Autodesk Fusion 360 part; units mm, degrees
(part 2 of 3)
sketch "gears_laser_cut" plane through (0, 0, 0) normal (1, 0, 0) x (0, 0, -1)
  arc A0 (348.8153, 272.0785) -> (348.6305, 272.3491) centre (348.5669, 272.1073) ccw
  arc A1 (349.0339, 271.6922) -> (348.78, 271.7745) centre (344.1421, 257.037) ccw
  arc A2 (342.0659, 272.3469) -> (341.8017, 272.3087) centre (344.1421, 257.037) ccw
  arc A3 (345.287, 272.746) -> (345.0457, 272.9677) centre (345.0386, 272.7178) ccw
  arc A4 (347.0702, 272.5131) -> (346.8558, 272.7609) centre (346.8202, 272.5134) ccw
  line L0 (365.4314, 255.9231) -> (365.9486, 256.0584)
  line L1 (387.4886, 271.4519) -> (387.367, 270.9313)
  line L2 (387.305, 271.7538) -> (387.3359, 271.7418)
  line L3 (348.5984, 272.3575) -> (347.7859, 272.5711)
  line L4 (365.2501, 255.6199) -> (365.3445, 254.7966)
  line L5 (365.4024, 256.3282) -> (365.9379, 256.2419)
  line L6 (343.1909, 272.964) -> (343.2239, 272.9669)
  line L7 (369.0501, 267.4461) -> (368.5255, 266.8046)
  line L8 (386.5329, 272.0545) -> (386.4983, 272.0679)
  line L9 (370.3154, 268.7566) -> (370.3392, 268.7797)
  arc A5 (382.3711, 241.8617) -> (382.5542, 241.8777) centre (381.1421, 257.037) ccw
  arc A6 (349.4983, 272.0679) -> (349.1921, 271.9615) centre (349.4076, 271.8349) ccw
  line L10 (365.1921, 257.4407) -> (365.1921, 256.612)
  arc A7 (343.4888, 272.7741) -> (343.2239, 272.9669) centre (343.2452, 272.7178) ccw
  arc A8 (349.2026, 242.1214) -> (349.5112, 242.0112) centre (349.4205, 242.2441) ccw
  arc A9 (345.341, 241.6336) -> (345.6069, 241.6566) centre (344.1421, 257.037) ccw
  line L11 (387.8604, 271.2886) -> (387.5342, 270.8552)
  arc A10 (345.5874, 272.4193) -> (345.3215, 272.4419) centre (344.1421, 257.037) ccw
  arc A11 (382.0595, 241.1067) -> (382.3002, 241.324) centre (382.0523, 241.3566) ccw
  arc A12 (346.8694, 241.3151) -> (347.0838, 241.5584) centre (346.8338, 241.5626) ccw
  arc A13 (340.3342, 272.0104) -> (340.0761, 271.9424) centre (344.1421, 257.037) ccw
  line L12 (369.6642, 267.8305) -> (369.9756, 267.3863)
  arc A14 (342.3169, 272.889) -> (342.0889, 272.6584) centre (342.3382, 272.6399) ccw
  arc A15 (341.6992, 272.5971) -> (341.414, 272.7584) centre (341.4636, 272.5133) ccw
  arc A16 (340.5218, 272.5776) -> (340.3216, 272.3225) centre (340.5714, 272.3326) ccw
  arc A17 (344.1357, 272.9937) -> (343.883, 272.7906) centre (344.1286, 272.7438) ccw
  line L13 (370.3154, 268.7566) -> (369.7212, 268.1791)
  line L14 (388.2096, 271.3421) -> (388.1768, 271.3594)
  arc A18 (348.7987, 242.3055) -> (349.0524, 242.3881) centre (344.1421, 257.037) ccw
  line L15 (348.5984, 272.3575) -> (348.6305, 272.3491)
  arc A19 (380.9075, 241.2886) -> (381.161, 241.0811) centre (381.1539, 241.331) ccw
  line L16 (347.4579, 272.4399) -> (347.3315, 272.1543)
  arc A20 (345.9547, 272.8904) -> (345.6805, 272.7174) centre (345.9191, 272.643) ccw
  arc A21 (347.75, 272.5805) -> (347.4579, 272.4399) centre (347.6865, 272.3387) ccw
  arc A22 (384.0929, 242.1007) -> (384.273, 242.1374) centre (381.1421, 257.037) ccw
  arc A23 (384.4805, 241.6447) -> (384.7745, 241.5) centre (384.7109, 241.7418) ccw
  arc A24 (347.4694, 241.6418) -> (347.7633, 241.4971) centre (347.6998, 241.7389) ccw
  arc A25 (382.7042, 241.3645) -> (382.9797, 241.1872) centre (382.9442, 241.4347) ccw
  line L17 (369.7212, 268.1791) -> (369.6946, 268.1533)
  line L18 (343.883, 272.7906) -> (343.8246, 272.4838)
  line L19 (369.3939, 267.5274) -> (369.8514, 267.2508)
  arc A26 (380.2376, 241.106) -> (380.5015, 241.2944) centre (380.2589, 241.3551) ccw
  line L20 (341.3815, 272.7518) -> (341.414, 272.7584)
  line L21 (369.0501, 267.4461) -> (369.071, 267.4717)
  line L22 (347.0838, 241.5584) -> (347.089, 241.8707)
  line L23 (387.305, 271.7538) -> (386.5329, 272.0545)
  arc A27 (343.8246, 272.4838) -> (343.5578, 272.476) centre (344.1421, 257.037) ccw
  line L24 (345.0126, 272.9687) -> (345.0457, 272.9677)
  arc A28 (347.3315, 272.1543) -> (347.0698, 272.2071) centre (344.1421, 257.037) ccw
  arc A29 (345.0595, 241.1067) -> (345.3002, 241.324) centre (345.0523, 241.3566) ccw
  line L25 (348.608, 241.7191) -> (348.6438, 241.7285)
  line L26 (365.2501, 255.6199) -> (365.2463, 255.6528)
  line L27 (384.8065, 241.5084) -> (384.7745, 241.5)
  arc A30 (347.089, 241.8707) -> (347.3506, 241.9238) centre (344.1421, 257.037) ccw
  arc A31 (339.9414, 272.2172) -> (339.6397, 272.3449) centre (339.7169, 272.1071) ccw
  line L28 (365.1921, 256.612) -> (365.1921, 256.575)
  arc A32 (383.8694, 241.3151) -> (384.0838, 241.5584) centre (383.8338, 241.5626) ccw
  line L29 (346.823, 272.7656) -> (346.8558, 272.7609)
  arc A33 (380.6332, 241.8205) -> (380.8169, 241.8155) centre (381.1421, 257.037) ccw
  line L30 (347.0702, 272.5131) -> (347.0698, 272.2071)
  arc A34 (345.6928, 241.3629) -> (345.9683, 241.1856) centre (345.9327, 241.433) ccw
  line L31 (349.542, 242.0232) -> (349.5112, 242.0112)
  arc A35 (348.6438, 241.7285) -> (348.829, 241.9946) centre (348.5802, 241.9703) ccw
  line L32 (342.0889, 272.6584) -> (342.0659, 272.3469)
  line L33 (347.4694, 241.6418) -> (347.3506, 241.9238)
  line L34 (345.6805, 272.7174) -> (345.5874, 272.4193)
  line L35 (346.8327, 241.3099) -> (346.8694, 241.3151)
  line L36 (343.4888, 272.7741) -> (343.5578, 272.476)
  line L37 (365.3445, 254.7966) -> (365.3488, 254.7598)
  line L38 (384.4805, 241.6447) -> (384.273, 242.1374)
  line L39 (368.5255, 266.8046) -> (368.5021, 266.7759)
  line L40 (369.7365, 245.8801) -> (369.7128, 245.9032)
  line L41 (395.196, 249.9145) -> (394.7721, 250.2529)
  arc A36 (368.7814, 248.1481) -> (368.8896, 247.9996) centre (381.1421, 257.037) ccw
  line L42 (359.7722, 255.0515) -> (359.4768, 255.153)
  line L43 (395.9995, 251.2197) -> (396.0139, 251.2538)
  arc A37 (365.9644, 261.9618) -> (366.0795, 261.6587) centre (366.1999, 261.8778) ccw
  arc A38 (365.9464, 257.9803) -> (365.9361, 257.7968) centre (381.1421, 257.037) ccw
  line L44 (359.3291, 252.145) -> (359.3197, 252.1133)
  arc A39 (367.8487, 249.6151) -> (367.9393, 249.4552) centre (381.1421, 257.037) ccw
  line L45 (355.2589, 268.2021) -> (354.9982, 268.0302)
  line L46 (359.3291, 252.145) -> (359.5658, 252.9512)
  arc A40 (366.7194, 250.7083) -> (366.6359, 250.3915) centre (366.8603, 250.5018) ccw
  arc A41 (365.5874, 259.5105) -> (365.3459, 259.2891) centre (365.5943, 259.2606) ccw
  arc A42 (368.5276, 247.6061) -> (368.5181, 247.2786) centre (368.7116, 247.4369) ccw
  line L47 (359.5283, 253.6682) -> (359.2224, 253.6773)
  line L48 (360.0424, 255.712) -> (360.0405, 255.6789)
  line L49 (359.044, 251.9363) -> (358.7411, 251.9802)
  arc A43 (366.5549, 261.3976) -> (366.5033, 261.2211) centre (381.1421, 257.037) ccw
  arc A44 (392.9753, 266.6171) -> (392.8587, 266.7592) centre (381.1421, 257.037) ccw
  line L50 (332.0574, 267.455) -> (332.0783, 267.4806)
  line L51 (358.6724, 250.4457) -> (358.9995, 251.2197)
  line L52 (354.9009, 268.8194) -> (354.926, 268.7977)
  line L53 (396.0472, 251.9473) -> (395.5182, 252.024)
  arc A45 (365.9707, 261.2675) -> (365.7056, 261.0751) centre (365.9491, 261.0184) ccw
  line L54 (356.7961, 266.756) -> (356.7744, 266.786)
  arc A46 (391.8061, 267.9035) -> (391.6741, 268.0315) centre (381.1421, 257.037) ccw
  line L55 (395.9163, 251.563) -> (395.4566, 251.8508)
  line L56 (395.6769, 250.4564) -> (395.664, 250.4259)
  line L57 (359.812, 255.4441) -> (359.5071, 255.4182)
  line L58 (332.4012, 267.5363) -> (332.6631, 267.378)
  arc A47 (391.9637, 268.4809) -> (391.9172, 268.8052) centre (391.7535, 268.6163) ccw
  arc A48 (367.5348, 249.1055) -> (367.488, 248.7812) centre (367.6983, 248.9164) ccw
  line L59 (359.7877, 253.9081) -> (359.7821, 253.8755)
  line L60 (395.2395, 249.564) -> (395.2577, 249.5962)
  arc A49 (365.2434, 258.3962) -> (365.4242, 258.127) centre (365.4918, 258.3677) ccw
  arc A50 (365.502, 260.1996) -> (365.6509, 259.9116) centre (365.7455, 260.143) ccw
  arc A51 (369.6849, 246.2296) -> (369.7128, 245.9032) centre (369.887, 246.0825) ccw
  line L61 (354.9724, 268.4733) -> (354.8066, 268.2161)
  line L62 (356.1739, 267.5161) -> (355.6058, 268.1351)
  arc A52 (393.9902, 265.2058) -> (393.8906, 265.3603) centre (381.1421, 257.037) ccw
  arc A53 (358.6516, 251.7287) -> (358.7411, 251.9802) centre (344.1421, 257.037) ccw
  arc A54 (369.8752, 246.7971) -> (369.9996, 246.6618) centre (381.1421, 257.037) ccw
  line L63 (358.3654, 250.2708) -> (358.0695, 250.349)
  line L64 (369.6849, 246.2296) -> (369.9996, 246.6618)
  arc A55 (367.9739, 248.0251) -> (368.2843, 247.9312) centre (368.1842, 248.1603) ccw
  arc A56 (369.0871, 246.5828) -> (369.4061, 246.5248) centre (369.2806, 246.741) ccw
  line L65 (357.8215, 265.2502) -> (357.8033, 265.2825)
  arc A57 (367.0325, 249.5849) -> (367.3301, 249.4562) centre (367.2568, 249.6952) ccw
  line L66 (358.196, 249.9145) -> (357.9519, 250.1094)
  line L67 (358.9995, 251.2197) -> (359.0139, 251.2538)
  arc A58 (366.1529, 259.7063) -> (366.1218, 259.5252) centre (381.1421, 257.037) ccw
  line L68 (359.7877, 253.9081) -> (359.931, 254.736)
  line L69 (359.5658, 252.9512) -> (359.5762, 252.9867)
  line L70 (358.2395, 249.564) -> (358.2577, 249.5962)
  line L71 (395.6769, 250.4564) -> (395.9995, 251.2197)
  arc A59 (366.275, 251.2419) -> (366.556, 251.0801) centre (366.5104, 251.3259) ccw
  line L72 (369.4061, 246.5248) -> (369.8752, 246.7971)
  line L73 (369.7365, 245.8801) -> (370.3308, 245.3026)
  line L74 (358.9163, 251.563) -> (358.6516, 251.7287)
  line L75 (358.6686, 263.6374) -> (358.6542, 263.6715)
  arc A60 (367.0893, 251.1788) -> (367.161, 251.0096) centre (381.1421, 257.037) ccw
  line L76 (358.6724, 250.4457) -> (358.6595, 250.4152)
  line L77 (395.3699, 250.2815) -> (394.853, 250.418)
  line L78 (359.444, 253.2828) -> (359.1621, 253.4173)
  arc A61 (395.3699, 250.2815) -> (395.664, 250.4259) centre (395.4337, 250.5232) ccw
  line L79 (333.3237, 268.7646) -> (333.3475, 268.7877)
  arc A62 (359.1621, 253.4173) -> (359.2224, 253.6773) centre (344.1421, 257.037) ccw
  line L80 (391.8922, 268.8269) -> (391.9172, 268.8052)
  line L81 (396.5658, 252.9512) -> (396.5762, 252.9867)
  arc A63 (393.7744, 266.786) -> (393.4592, 266.8621) centre (393.5721, 266.6391) ccw
  arc A64 (394.8033, 265.2825) -> (394.4989, 265.394) centre (394.5856, 265.1596) ccw
  arc A65 (358.3654, 250.2708) -> (358.6595, 250.4152) centre (358.4293, 250.5126) ccw
  arc A66 (393.1976, 267.1727) -> (393.1885, 267.5002) centre (393.0043, 267.3312) ccw
  arc A67 (359.812, 255.4441) -> (360.0405, 255.6789) centre (359.7909, 255.6932) ccw
  line L82 (332.6642, 267.8305) -> (332.8435, 267.5747)
  line L83 (331.5086, 266.4517) -> (331.7159, 266.2181)
  arc A68 (394.2744, 265.7324) -> (394.3027, 266.0589) centre (394.1004, 265.9119) ccw
  line L84 (330.5178, 264.9502) -> (330.7503, 264.7418)
  line L85 (330.9486, 266.0095) -> (330.9665, 266.0374)
  arc A69 (359.4768, 255.153) -> (359.5071, 255.4182) centre (344.1421, 257.037) ccw
  line L86 (392.2589, 268.2021) -> (391.8061, 267.9035)
  arc A70 (359.9373, 254.7725) -> (359.7722, 255.0515) centre (359.691, 254.8151) ccw
  line L87 (392.6058, 268.1351) -> (392.5807, 268.1624)
  line L88 (393.1661, 267.5246) -> (392.6058, 268.1351)
  line L89 (396.8127, 255.4556) -> (396.28, 255.4104)
  line L90 (357.29, 266.0763) -> (357.3094, 266.0495)
  arc A71 (357.9519, 250.1094) -> (358.0695, 250.349) centre (344.1421, 257.037) ccw
  line L91 (357.4989, 265.394) -> (357.2059, 265.2856)
  arc A72 (359.044, 251.9363) -> (359.3197, 252.1133) centre (359.0799, 252.1837) ccw
  line L92 (396.444, 253.2828) -> (395.9545, 253.5164)
  line L93 (355.6058, 268.1351) -> (355.5807, 268.1624)
  arc A73 (359.5283, 253.6682) -> (359.7821, 253.8755) centre (359.5357, 253.9181) ccw
  line L94 (396.7897, 253.9195) -> (396.784, 253.8868)
  line L95 (330.0118, 264.4471) -> (330.0264, 264.4768)
  line L96 (397.0431, 255.7235) -> (397.0904, 256.5508)
  arc A74 (359.5762, 252.9867) -> (359.444, 253.2828) centre (359.3363, 253.0572) ccw
  line L97 (330.9486, 266.0095) -> (330.4944, 265.3027)
  arc A75 (392.5807, 268.1624) -> (392.2589, 268.2021) centre (392.3965, 267.9934) ccw
  arc A76 (358.2577, 249.5962) -> (358.196, 249.9145) centre (358.04, 249.7191) ccw
  line L98 (393.1661, 267.5246) -> (393.1885, 267.5002)
  line L99 (356.1739, 267.5161) -> (356.1963, 267.4917)
  line L100 (391.8922, 268.8269) -> (391.2659, 269.3696)
  line L101 (358.3644, 263.817) -> (358.0611, 263.7427)
  line L102 (357.29, 266.0763) -> (356.7961, 266.756)
  arc A77 (395.2577, 249.5962) -> (395.196, 249.9145) centre (395.04, 249.7191) ccw
  line L103 (333.9693, 269.0685) -> (334.1183, 268.794)
  line L104 (396.7897, 253.9195) -> (396.931, 254.736)
  line L105 (358.2347, 264.5187) -> (358.251, 264.4898)
  line L106 (357.2812, 265.7231) -> (357.0615, 265.5101)
  line L107 (391.9637, 268.4809) -> (391.6741, 268.0315)
  arc A78 (359.0139, 251.2538) -> (358.9163, 251.563) centre (358.7836, 251.3511) ccw
  line L108 (332.0574, 267.455) -> (331.5255, 266.8046)
  line L109 (331.2809, 266.1295) -> (331.5592, 266.0021)
  line L110 (396.5303, 253.6796) -> (395.9959, 253.6955)
  line L111 (356.4592, 266.8621) -> (356.1805, 266.721)
  line L112 (330.0118, 264.4471) -> (329.6411, 263.6931)
  line L113 (396.931, 254.736) -> (396.9373, 254.7725)
  line L114 (396.3323, 252.1561) -> (396.323, 252.1243)
  line L115 (333.6746, 268.8062) -> (333.9167, 268.6191)
  line L116 (333.3237, 268.7646) -> (332.7212, 268.1791)
  line L117 (397.0431, 255.7235) -> (397.0412, 255.6904)
  line L118 (393.1976, 267.1727) -> (392.8587, 266.7592)
  line L119 (396.3323, 252.1561) -> (396.5658, 252.9512)
  line L120 (358.1857, 264.1687) -> (357.9431, 263.9821)
  line L121 (358.2347, 264.5187) -> (357.8215, 265.2502)
  line L122 (396.7722, 255.0515) -> (396.2592, 255.2278)
  line L123 (330.3283, 264.6042) -> (330.6192, 264.5093)
  line L124 (356.2054, 267.1642) -> (356.0114, 266.9275)
  arc A79 (358.1857, 264.1687) -> (358.251, 264.4898) centre (358.0333, 264.3669) ccw
  line L125 (371.7219, 269.9144) -> (371.0657, 269.4083)
  line L126 (372.5599, 243.5867) -> (372.5316, 243.6038)
  arc A80 (330.3283, 264.6042) -> (330.0264, 264.4768) centre (330.2508, 264.3665) ccw
  arc A81 (354.9724, 268.4733) -> (354.926, 268.7977) centre (354.7622, 268.6087) ccw
  arc A82 (396.2592, 255.2278) -> (396.28, 255.4104) centre (381.1421, 257.037) ccw
  arc A83 (331.2809, 266.1295) -> (330.9665, 266.0374) centre (331.1768, 265.9022) ccw
  line L127 (372.0753, 269.9157) -> (372.4582, 269.5426)
  line L128 (371.7219, 269.9144) -> (371.7482, 269.9346)
  arc A84 (375.6876, 271.2514) -> (375.5164, 271.1845) centre (381.1421, 257.037) ccw
  line L129 (394.2832, 266.0857) -> (394.3027, 266.0589)
  line L130 (334.0657, 269.4083) -> (334.0364, 269.3857)
  arc A85 (396.5303, 253.6796) -> (396.784, 253.8868) centre (396.5377, 253.9295) ccw
  line L131 (332.7212, 268.1791) -> (332.6946, 268.1533)
  arc A86 (356.7744, 266.786) -> (356.4592, 266.8621) centre (356.5721, 266.6391) ccw
  arc A87 (396.8127, 255.4556) -> (397.0412, 255.6904) centre (396.7916, 255.7047) ccw
  line L132 (394.8215, 265.2502) -> (394.8033, 265.2825)
  line L133 (394.2832, 266.0857) -> (393.7961, 266.756)
  arc A88 (372.0753, 269.9157) -> (371.7482, 269.9346) centre (371.9008, 269.7366) ccw
  line L134 (370.9915, 244.9941) -> (371.255, 245.4593)
  line L135 (371.0827, 244.6527) -> (371.0564, 244.6729)
  arc A89 (375.7739, 272.0636) -> (375.6041, 271.7874) centre (375.8511, 271.8258) ccw
  line L136 (371.7389, 244.1467) -> (371.7682, 244.124)
  arc A90 (396.0472, 251.9473) -> (396.323, 252.1243) centre (396.0831, 252.1948) ccw
  line L137 (370.3308, 245.3026) -> (370.3573, 245.2768)
  arc A91 (333.6746, 268.8062) -> (333.3475, 268.7877) centre (333.5217, 268.6084) ccw
  arc A92 (394.7721, 250.2529) -> (394.853, 250.418) centre (381.1421, 257.037) ccw
  arc A93 (330.4743, 265.2716) -> (330.5178, 264.9502) centre (330.6846, 265.1364) ccw
  arc A94 (395.4566, 251.8508) -> (395.5182, 252.024) centre (381.1421, 257.037) ccw
  line L138 (330.4944, 265.3027) -> (330.4743, 265.2716)
  arc A95 (358.0611, 263.7427) -> (357.9431, 263.9821) centre (344.1421, 257.037) ccw
  arc A96 (356.1805, 266.721) -> (356.0114, 266.9275) centre (344.1421, 257.037) ccw
  arc A97 (358.6542, 263.6715) -> (358.3644, 263.817) centre (358.4239, 263.5742) ccw
  arc A98 (355.5807, 268.1624) -> (355.2589, 268.2021) centre (355.3965, 267.9934) ccw
  arc A99 (374.096, 271.3537) -> (373.9588, 271.0599) centre (374.1998, 271.1263) ccw
  arc A100 (357.2059, 265.2856) -> (357.0615, 265.5101) centre (344.1421, 257.037) ccw
  line L139 (393.7961, 266.756) -> (393.7744, 266.786)
  line L140 (370.6809, 245.2555) -> (371.1159, 245.5795)
  line L141 (394.4989, 265.394) -> (393.9902, 265.2058)
  arc A101 (357.2812, 265.7231) -> (357.3094, 266.0495) centre (357.1072, 265.9026) ccw
  line L142 (372.4582, 269.5426) -> (372.6098, 269.6466)
  arc A102 (396.0139, 251.2538) -> (395.9163, 251.563) centre (395.7836, 251.3511) ccw
  arc A103 (375.2279, 271.6346) -> (374.9136, 271.7271) centre (375.0174, 271.4997) ccw
  line L143 (394.2744, 265.7324) -> (393.8906, 265.3603)
  arc A104 (332.4012, 267.5363) -> (332.0783, 267.4806) centre (332.2719, 267.3224) ccw
  arc A105 (395.9545, 253.5164) -> (395.9959, 253.6955) centre (381.1421, 257.037) ccw
  arc A106 (396.9373, 254.7725) -> (396.7722, 255.0515) centre (396.691, 254.8151) ccw
  arc A107 (372.5099, 270.4572) -> (372.4071, 270.1497) centre (372.639, 270.2431) ccw
  arc A108 (373.6024, 270.8653) -> (373.2796, 270.9213) centre (373.4087, 270.7072) ccw
  line L144 (371.0827, 244.6527) -> (371.7389, 244.1467)
  line L145 (372.092, 244.1398) -> (372.4873, 244.5113)
  circle A109 centre (381.1421, 257.037) radius 3.75
  arc A110 (356.2054, 267.1642) -> (356.1963, 267.4917) centre (356.0121, 267.3227) ccw
  arc A111 (357.8033, 265.2825) -> (357.4989, 265.394) centre (357.5856, 265.1596) ccw
  arc A112 (330.7503, 264.7418) -> (330.6192, 264.5093) centre (344.1421, 257.037) ccw
  line L146 (393.4592, 266.8621) -> (392.9753, 266.6171)
  arc A113 (354.9982, 268.0302) -> (354.8066, 268.2161) centre (344.1421, 257.037) ccw
  line L147 (358.9957, 262.8635) -> (358.6686, 263.6374)
  line L148 (373.9404, 270.451) -> (374.1028, 270.537)
  line L149 (331.5255, 266.8046) -> (331.5021, 266.7759)
  arc A114 (396.5762, 252.9867) -> (396.444, 253.2828) centre (396.3363, 253.0572) ccw
  arc A115 (331.7159, 266.2181) -> (331.5592, 266.0021) centre (344.1421, 257.037) ccw
  arc A116 (332.8435, 267.5747) -> (332.6631, 267.378) centre (344.1421, 257.037) ccw
  line L150 (372.4305, 243.9155) -> (372.6392, 244.4077)
  line L151 (395.6686, 263.6374) -> (395.6542, 263.6715)
  line L152 (354.2734, 244.7109) -> (354.2484, 244.6893)
  line L153 (374.1491, 242.6961) -> (374.119, 242.7098)
  line L154 (389.8118, 243.6429) -> (390.4958, 244.1107)
  line L155 (354.9852, 245.6059) -> (354.8208, 245.8715)
  line L156 (373.2695, 243.1588) -> (373.3013, 243.1397)
  line L157 (373.9588, 271.0599) -> (374.1028, 270.537)
  line L158 (373.6212, 243.1923) -> (373.9716, 243.6063)
  line L159 (373.983, 243.008) -> (374.1342, 243.5207)
  arc A117 (370.9915, 244.9941) -> (371.0564, 244.6729) centre (371.2091, 244.8709) ccw
  line L160 (390.4958, 244.1107) -> (390.5264, 244.1316)
  line L161 (374.8834, 271.7133) -> (374.9136, 271.7271)
  line L162 (374.1297, 271.3691) -> (374.096, 271.3537)
  line L163 (356.1805, 246.5652) -> (356.2056, 246.5924)
  arc A118 (373.983, 243.008) -> (374.119, 242.7098) centre (374.2228, 242.9372) ccw
  arc A119 (396.3159, 261.974) -> (396.0446, 262.1516) centre (396.076, 261.9036) ccw
  line L164 (357.8264, 248.8324) -> (357.8101, 248.8035)
  line L165 (395.229, 264.5287) -> (394.8215, 265.2502)
  line L166 (373.2512, 270.9042) -> (372.5416, 270.4763)
  line L167 (356.2176, 246.9165) -> (356.0239, 247.1616)
  line L168 (395.9912, 262.8741) -> (395.6686, 263.6374)
  line L169 (353.4958, 244.1107) -> (353.5264, 244.1316)
  line L170 (372.5599, 243.5867) -> (373.2695, 243.1588)
  line L171 (374.8834, 271.7133) -> (374.1297, 271.3691)
  line L172 (373.2512, 270.9042) -> (373.2796, 270.9213)
  arc A120 (372.4873, 244.5113) -> (372.6392, 244.4077) centre (381.1421, 257.037) ccw
  line L173 (372.5416, 270.4763) -> (372.5099, 270.4572)
  line L174 (395.9912, 262.8741) -> (396.0041, 262.8436)
  arc A121 (371.1159, 245.5795) -> (371.255, 245.4593) centre (381.1421, 257.037) ccw
  line L175 (357.8264, 248.8324) -> (358.2395, 249.564)
  line L176 (375.8091, 272.075) -> (375.7739, 272.0636)
  line L177 (372.4071, 270.1497) -> (372.6098, 269.6466)
  arc A122 (334.0364, 269.3857) -> (333.9693, 269.0685) centre (334.1891, 269.1877) ccw
  line L178 (374.1491, 242.6961) -> (374.9029, 242.3518)
  line L179 (357.2925, 248.3589) -> (357.0722, 248.5803)
  arc A123 (331.5021, 266.7759) -> (331.5086, 266.4517) centre (331.6956, 266.6176) ccw
  arc A124 (371.7682, 244.124) -> (372.092, 244.1398) centre (371.9209, 244.322) ccw
  line L180 (353.9207, 244.6894) -> (353.6897, 244.8901)
  arc A125 (395.9026, 262.532) -> (396.0041, 262.8436) centre (395.7738, 262.7463) ccw
  line L181 (395.229, 264.5287) -> (395.2453, 264.4999)
  arc A126 (395.6542, 263.6715) -> (395.3644, 263.817) centre (395.4239, 263.5742) ccw
  arc A127 (395.5065, 262.0834) -> (395.4445, 262.2565) centre (381.1421, 257.037) ccw
  arc A128 (332.6946, 268.1533) -> (332.6642, 267.8305) centre (332.8689, 267.974) ccw
  arc A129 (372.4305, 243.9155) -> (372.5316, 243.6038) centre (372.6607, 243.8179) ccw
  arc A130 (373.3013, 243.1397) -> (373.6212, 243.1923) centre (373.4304, 243.3538) ccw
  line L182 (357.5014, 248.6936) -> (357.2164, 248.805)
  arc A131 (394.8376, 263.6879) -> (394.7563, 263.8528) centre (381.1421, 257.037) ccw
  arc A132 (334.1183, 268.794) -> (333.9167, 268.6191) centre (344.1421, 257.037) ccw
  line L183 (375.6041, 271.7874) -> (375.6876, 271.2514)
  arc A133 (370.3573, 245.2768) -> (370.6809, 245.2555) centre (370.5316, 245.456) ccw
  arc A134 (395.18, 264.1788) -> (395.2453, 264.4999) centre (395.0276, 264.3769) ccw
  line L184 (354.9084, 245.2612) -> (354.9363, 245.2854)
  line L185 (353.6115, 244.4444) -> (353.4784, 244.727)
  arc A135 (373.9716, 243.6063) -> (374.1342, 243.5207) centre (381.1421, 257.037) ccw
  line L186 (355.6124, 245.9462) -> (355.59, 245.9218)
  line L187 (375.2279, 271.6346) -> (375.5164, 271.1845)
  line L188 (354.2734, 244.7109) -> (354.9084, 245.2612)
  line L189 (373.6024, 270.8653) -> (373.9404, 270.451)
  line L190 (395.18, 264.1788) -> (394.7563, 263.8528)
  line L191 (355.2645, 245.8846) -> (355.0121, 246.0576)
  line L192 (357.2958, 248.0057) -> (357.3175, 248.0357)
  line L193 (395.3644, 263.817) -> (394.8376, 263.6879)
  line L194 (355.6124, 245.9462) -> (356.1805, 246.5652)
  line L195 (328.7007, 261.054) -> (328.5104, 260.2357)
  arc A136 (358.7347, 262.1123) -> (358.6449, 262.3637) centre (344.1421, 257.037) ccw
  arc A137 (359.4361, 260.8026) -> (359.5723, 261.1005) centre (359.3325, 261.0301) ccw
  line L196 (328.3434, 259.2677) -> (328.2476, 258.4329)
  arc A138 (396.7636, 259.046) -> (396.933, 259.3265) centre (396.6867, 259.2839) ccw
  line L197 (379.1138, 241.418) -> (379.0839, 241.9518)
  line L198 (397.0904, 256.5508) -> (397.0925, 256.5878)
  arc A139 (359.5916, 256.9133) -> (359.5915, 257.1803) centre (344.1421, 257.037) ccw
  line L199 (376.6175, 241.7363) -> (376.6527, 241.7249)
  line L200 (359.9293, 259.3478) -> (359.935, 259.3151)
  line L201 (379.0889, 272.6584) -> (379.0489, 272.1174)
  arc A140 (390.5264, 244.1316) -> (390.6115, 244.4444) centre (390.3853, 244.3379) ccw
  line L202 (359.8157, 258.6433) -> (359.505, 258.6753)
  line L203 (394.5071, 248.7037) -> (394.0091, 248.8982)
  line L204 (358.9957, 262.8635) -> (359.0086, 262.833)
  arc A141 (390.9294, 244.697) -> (391.2571, 244.6968) centre (391.0934, 244.8857) ccw
  line L205 (377.579, 241.4849) -> (378.3912, 241.3203)
  arc A142 (391.9363, 245.2854) -> (391.9852, 245.6059) centre (391.7726, 245.4743) ccw
  line L206 (329.2592, 262.788) -> (329.2704, 262.8192)
  line L207 (378.3912, 241.3203) -> (378.4275, 241.313)
  arc A143 (392.2723, 245.8931) -> (392.5978, 245.9303) centre (392.4136, 246.0993) ccw
  line L208 (375.8294, 241.9924) -> (375.7979, 242.0026)
  line L209 (379.3537, 272.8921) -> (379.3169, 272.889)
  arc A144 (396.2762, 258.6988) -> (396.255, 258.8814) centre (381.1421, 257.037) ccw
  line L210 (394.2925, 248.3589) -> (393.9099, 248.7434)
  line L211 (358.9071, 262.5214) -> (358.6449, 262.3637)
  line L212 (328.5887, 259.522) -> (328.8946, 259.5304)
  line L213 (371.0657, 269.4083) -> (371.0364, 269.3857)
  line L214 (359.0446, 262.1516) -> (358.7347, 262.1123)
  arc A145 (392.8813, 247.3421) -> (392.9975, 247.4845) centre (381.1421, 257.037) ccw
  arc A146 (393.2056, 246.5924) -> (393.2176, 246.9165) centre (393.0214, 246.7615) ccw
  line L215 (328.6509, 259.9116) -> (328.94, 259.7934)
  line L216 (378.6879, 272.5948) -> (378.867, 272.0911)
  arc A147 (396.7797, 260.2121) -> (396.5305, 260.4195) centre (396.5334, 260.1695) ccw
  arc A148 (393.9099, 248.7434) -> (394.0091, 248.8982) centre (381.1421, 257.037) ccw
  arc A149 (395.9881, 260.4131) -> (395.9462, 260.5921) centre (381.1421, 257.037) ccw
  line L217 (370.9693, 269.0685) -> (371.2281, 268.5918)
  arc A150 (359.505, 258.6753) -> (359.4744, 258.9404) centre (344.1421, 257.037) ccw
  arc A151 (393.47, 247.2345) -> (393.7892, 247.3085) centre (393.587, 247.4555) ccw
  line L218 (370.6663, 268.7982) -> (371.0893, 268.4712)
  line L219 (328.9734, 261.2787) -> (329.2782, 261.2522)
  line L220 (377.3466, 241.751) -> (377.3778, 242.2847)
  line L221 (375.8294, 241.9924) -> (376.6175, 241.7363)
  line L222 (376.9525, 241.8486) -> (377.1999, 242.3313)
  arc A152 (371.2281, 268.5918) -> (371.0893, 268.4712) centre (381.1421, 257.037) ccw
  line L223 (378.7111, 241.47) -> (378.902, 241.9777)
  arc A153 (394.3175, 248.0357) -> (394.2925, 248.3589) centre (394.1153, 248.1826) ccw
  line L224 (329.0795, 261.6587) -> (329.3533, 261.5083)
  arc A154 (397.0397, 258.4089) -> (396.8157, 258.6433) centre (396.7901, 258.3946) ccw
  line L225 (328.4242, 258.127) -> (328.7249, 258.0425)
  line L226 (379.375, 241.1801) -> (379.342, 241.1829)
  arc A155 (371.0364, 269.3857) -> (370.9693, 269.0685) centre (371.1891, 269.1877) ccw
  arc A156 (359.7656, 259.0346) -> (359.935, 259.3151) centre (359.6886, 259.2725) ccw
  line L227 (380.1794, 272.9631) -> (379.3537, 272.8921)
  line L228 (329.5558, 262.9802) -> (329.8556, 262.9191)
  line L229 (394.832, 248.8424) -> (394.8158, 248.8136)
  line L230 (394.832, 248.8424) -> (395.2395, 249.564)
  line L231 (328.9769, 261.9967) -> (328.9644, 261.9618)
  line L232 (377.579, 241.4849) -> (377.5465, 241.4915)
  line L233 (329.7045, 263.3456) -> (329.9594, 263.165)
  arc A157 (396.3669, 256.9628) -> (396.3667, 257.1466) centre (381.1421, 257.037) ccw
  arc A158 (396.4328, 260.8136) -> (396.5691, 261.1116) centre (396.3292, 261.0412) ccw
  line L234 (359.7656, 259.0346) -> (359.4744, 258.9404)
  arc A159 (329.3533, 261.5083) -> (329.2782, 261.2522) centre (344.1421, 257.037) ccw
  arc A160 (359.7797, 260.2121) -> (359.5305, 260.4195) centre (359.5334, 260.1695) ccw
  line L235 (396.9273, 259.3591) -> (396.786, 260.1756)
  arc A161 (359.3159, 261.974) -> (359.0446, 262.1516) centre (359.076, 261.9036) ccw
  line L236 (396.5598, 261.1434) -> (396.5691, 261.1116)
  arc A162 (328.5887, 259.522) -> (328.3472, 259.3006) centre (328.5956, 259.2721) ccw
  arc A163 (394.5071, 248.7037) -> (394.8158, 248.8136) centre (394.5981, 248.9365) ccw
  arc A164 (377.1999, 242.3313) -> (377.3778, 242.2847) centre (381.1421, 257.037) ccw
  arc A165 (329.9594, 263.165) -> (329.8556, 262.9191) centre (344.1421, 257.037) ccw
  arc A166 (391.6997, 246.0671) -> (391.8313, 246.1954) centre (381.1421, 257.037) ccw
  arc A167 (329.5558, 262.9802) -> (329.2704, 262.8192) centre (329.5058, 262.7352) ccw
  arc A168 (328.4068, 257.7328) -> (328.1921, 257.4853) centre (328.4421, 257.4853) ccw
  line L237 (328.3434, 259.2677) -> (328.3472, 259.3006)
  circle A169 centre (344.1421, 257.037) radius 3.75
  arc A170 (328.7249, 258.0425) -> (328.7098, 257.776) centre (344.1421, 257.037) ccw
  arc A171 (328.9644, 261.9618) -> (329.0795, 261.6587) centre (329.1999, 261.8778) ccw
  line L238 (396.7636, 259.046) -> (396.255, 258.8814)
  line L239 (397.0892, 257.5446) -> (397.0418, 258.3719)
  arc A172 (329.275, 251.2419) -> (329.556, 251.0801) centre (329.5104, 251.3259) ccw
  arc A173 (328.94, 259.7934) -> (328.8946, 259.5304) centre (344.1421, 257.037) ccw
  arc A174 (328.8978, 254.5244) -> (328.9435, 254.2614) centre (344.1421, 257.037) ccw
  arc A175 (328.7108, 256.2785) -> (328.7262, 256.0121) centre (344.1421, 257.037) ccw
  line L240 (338.6179, 242.2869) -> (338.6705, 242.5884)
  arc A176 (377.3466, 241.751) -> (377.5465, 241.4915) centre (377.5962, 241.7365) ccw
  line L241 (336.9725, 243.0127) -> (337.0591, 243.3063)
  arc A177 (396.8908, 257.2522) -> (397.091, 257.5115) centre (396.8415, 257.4973) ccw
  line L242 (338.2484, 242.4252) -> (338.4217, 242.6851)
  line L243 (342.3636, 241.1811) -> (342.3306, 241.1839)
  arc A178 (375.6289, 242.2833) -> (375.7979, 242.0026) centre (375.8752, 242.2404) ccw
  line L244 (396.4328, 260.8136) -> (395.9462, 260.5921)
  line L245 (396.5305, 260.4195) -> (395.9881, 260.4131)
  arc A179 (358.9071, 262.5214) -> (359.0086, 262.833) centre (358.7783, 262.7356) ccw
  arc A180 (397.0925, 256.5878) -> (396.8967, 256.8462) centre (396.8429, 256.602) ccw
  line L246 (396.786, 260.1756) -> (396.7797, 260.2121)
  arc A181 (328.2434, 258.3962) -> (328.4242, 258.127) centre (328.4918, 258.3677) ccw
  line L247 (397.0892, 257.5446) -> (397.091, 257.5115)
  line L248 (379.375, 241.1801) -> (380.2007, 241.1092)
  arc A182 (359.2181, 260.4158) -> (359.1575, 260.6758) centre (344.1421, 257.037) ccw
  line L249 (396.8908, 257.2522) -> (396.3667, 257.1466)
  arc A183 (378.4275, 241.313) -> (378.7111, 241.47) centre (378.4771, 241.558) ccw
  line L250 (396.8967, 256.8462) -> (396.3669, 256.9628)
  arc A184 (375.5493, 242.8765) -> (375.7207, 242.81) centre (381.1421, 257.037) ccw
  arc A185 (378.902, 241.9777) -> (379.0839, 241.9518) centre (381.1421, 257.037) ccw
  arc A186 (360.0397, 258.4089) -> (359.8157, 258.6433) centre (359.7901, 258.3946) ccw
  arc A187 (328.502, 260.1996) -> (328.6509, 259.9116) centre (328.7455, 260.143) ccw
  arc A188 (329.6248, 263.6599) -> (329.7045, 263.3456) centre (329.8491, 263.5496) ccw
  line L251 (396.9273, 259.3591) -> (396.933, 259.3265)
  arc A189 (328.9734, 261.2787) -> (328.7082, 261.0863) centre (328.9517, 261.0297) ccw
  arc A190 (328.4301, 255.9346) -> (328.245, 255.6642) centre (328.4934, 255.6927) ccw
  line L252 (396.8157, 258.6433) -> (396.2762, 258.6988)
  arc A191 (331.5705, 248.0561) -> (331.7275, 247.8403) centre (344.1421, 257.037) ccw
  arc A192 (374.9365, 242.3365) -> (375.2484, 242.4252) centre (375.0404, 242.5639) ccw
  arc A193 (376.6527, 241.7249) -> (376.9525, 241.8486) centre (376.73, 241.9627) ccw
  arc A194 (359.8915, 257.2407) -> (360.0917, 257.5) centre (359.8421, 257.4858) ccw
  arc A195 (379.1138, 241.418) -> (379.342, 241.1829) centre (379.3634, 241.432) ccw
  arc A196 (330.0325, 249.5849) -> (330.3301, 249.4562) centre (330.2568, 249.6952) ccw
  line L253 (397.0418, 258.3719) -> (397.0397, 258.4089)
  arc A197 (390.3804, 244.9351) -> (390.5258, 245.0476) centre (381.1421, 257.037) ccw
  arc A198 (360.0925, 256.5878) -> (359.8967, 256.8462) centre (359.8429, 256.602) ccw
  line L254 (343.5015, 241.2944) -> (343.5773, 241.5974)
  line L255 (335.5501, 243.5927) -> (335.5217, 243.6098)
  arc A199 (341.4275, 241.313) -> (341.7111, 241.47) centre (341.4771, 241.558) ccw
  line L256 (337.1386, 242.7009) -> (337.9029, 242.3518)
  arc A200 (335.3197, 244.3537) -> (335.5401, 244.2032) centre (344.1421, 257.037) ccw
  arc A201 (333.9824, 245.0011) -> (334.0473, 244.6799) centre (334.2, 244.8779) ccw
  arc A202 (331.5203, 247.615) -> (331.5108, 247.2875) centre (331.7043, 247.4458) ccw
  line L257 (343.2007, 241.1092) -> (343.2376, 241.106)
  line L258 (342.1023, 241.419) -> (342.0852, 241.7246)
  arc A203 (343.5773, 241.5974) -> (343.8441, 241.5899) centre (344.1421, 257.037) ccw
  line L259 (340.5677, 241.4872) -> (340.5352, 241.4937)
  line L260 (334.0735, 244.6597) -> (334.7389, 244.1467)
  line L261 (344.1826, 241.0817) -> (344.1495, 241.0807)
  line L262 (338.8185, 241.996) -> (338.787, 242.0062)
  arc A204 (328.7113, 252.9744) -> (328.972, 252.7816) centre (328.9548, 253.031) ccw
  line L263 (335.5501, 243.5927) -> (336.2695, 243.1588)
  line L264 (334.7389, 244.1467) -> (334.7682, 244.124)
  line L265 (335.4206, 243.9214) -> (335.5401, 244.2032)
  arc A205 (338.6179, 242.2869) -> (338.787, 242.0062) centre (338.8642, 242.244) ccw
  arc A206 (342.1023, 241.419) -> (342.3306, 241.1839) centre (342.352, 241.433) ccw
  arc A207 (332.6762, 246.6816) -> (332.8568, 246.4851) centre (344.1421, 257.037) ccw
  line L266 (341.3912, 241.3203) -> (341.4275, 241.313)
  arc A208 (343.2376, 241.106) -> (343.5015, 241.2944) centre (343.2589, 241.3551) ccw
  arc A209 (332.6766, 246.2377) -> (332.7045, 245.9112) centre (332.8787, 246.0905) ccw
  arc A210 (333.9314, 245.4421) -> (334.1332, 245.2674) centre (344.1421, 257.037) ccw
  line L267 (336.2695, 243.1588) -> (336.3013, 243.1397)
  line L268 (337.1386, 242.7009) -> (337.1085, 242.7146)
  arc A211 (340.3353, 241.7533) -> (340.5352, 241.4937) centre (340.5849, 241.7388) ccw
  line L269 (328.3445, 254.7966) -> (328.3488, 254.7598)
  arc A212 (330.9739, 248.0251) -> (331.2843, 247.9312) centre (331.1842, 248.1603) ccw
  line L270 (328.4301, 255.9346) -> (328.7262, 256.0121)
  arc A213 (328.3488, 254.7598) -> (328.5858, 254.5386) centre (328.5971, 254.7883) ccw
  line L271 (340.3353, 241.7533) -> (340.3531, 242.0588)
  arc A214 (343.896, 241.2883) -> (344.1495, 241.0807) centre (344.1423, 241.3306) ccw
  arc A215 (339.6527, 241.7249) -> (339.9525, 241.8486) centre (339.73, 241.9627) ccw
  line L272 (328.1921, 256.612) -> (328.1921, 256.575)
  line L273 (341.7111, 241.47) -> (341.821, 241.7624)
  arc A216 (336.823, 243.4307) -> (337.0591, 243.3063) centre (344.1421, 257.037) ccw
  arc A217 (341.821, 241.7624) -> (342.0852, 241.7246) centre (344.1421, 257.037) ccw
  line L274 (336.6212, 243.1923) -> (336.823, 243.4307)
  arc A218 (328.6582, 254.1507) -> (328.5051, 253.861) centre (328.7486, 253.9177) ccw
  arc A219 (328.1921, 256.575) -> (328.4024, 256.3282) centre (328.4421, 256.575) ccw
  line L275 (342.3636, 241.1811) -> (343.2007, 241.1092)
  line L276 (343.896, 241.2883) -> (343.8441, 241.5899)
  line L277 (339.9525, 241.8486) -> (340.095, 242.1265)
  line L278 (337.9029, 242.3518) -> (337.9365, 242.3365)
  line L279 (328.1921, 257.4522) -> (328.1921, 256.612)
  line L280 (340.5677, 241.4872) -> (341.3912, 241.3203)
  line L281 (328.7029, 253.0104) -> (328.7113, 252.9744)
  arc A220 (335.4206, 243.9214) -> (335.5217, 243.6098) centre (335.6508, 243.8239) ccw
  line L282 (338.8185, 241.996) -> (339.6175, 241.7363)
  arc A221 (329.2836, 252.8031) -> (329.3589, 252.547) centre (344.1421, 257.037) ccw
  line L283 (344.1826, 241.0817) -> (345.0224, 241.1057)
  arc A222 (340.095, 242.1265) -> (340.3531, 242.0588) centre (344.1421, 257.037) ccw
  arc A223 (329.0881, 252.4045) -> (328.9691, 252.0993) centre (329.2045, 252.1833) ccw
  line L284 (328.4024, 256.3282) -> (328.7108, 256.2785)
  line L285 (328.5104, 260.2357) -> (328.502, 260.1996)
  line L286 (376.9304, 272.2136) -> (377.1657, 271.7336)
  arc A224 (354.8208, 245.8715) -> (355.0121, 246.0576) centre (344.1421, 257.037) ccw
  line L287 (359.3263, 261.9385) -> (359.3159, 261.974)
  line L288 (359.5305, 260.4195) -> (359.2181, 260.4158)
  line L289 (359.563, 261.1323) -> (359.3263, 261.9385)
  line L290 (393.8087, 247.3353) -> (393.7892, 247.3085)
  line L291 (356.8019, 247.326) -> (356.7824, 247.2992)
  line L292 (329.2592, 262.788) -> (328.9769, 261.9967)
  line L293 (360.0424, 255.712) -> (360.0904, 256.5508)
  line L294 (359.8915, 257.2407) -> (359.5915, 257.1803)
  line L295 (393.2176, 246.9165) -> (392.8813, 247.3421)
  line L296 (378.3702, 272.7495) -> (377.5581, 272.5849)
  arc A225 (377.3435, 271.7805) -> (377.1657, 271.7336) centre (381.1421, 257.037) ccw
  arc A226 (353.5264, 244.1316) -> (353.6115, 244.4444) centre (353.3853, 244.3379) ccw
  arc A227 (353.4784, 244.727) -> (353.6897, 244.8901) centre (344.1421, 257.037) ccw
  line L297 (374.9029, 242.3518) -> (374.9365, 242.3365)
  arc A228 (356.0239, 247.1616) -> (356.1928, 247.3683) centre (344.1421, 257.037) ccw
  arc A229 (378.6879, 272.5948) -> (378.4027, 272.7561) centre (378.4523, 272.5111) ccw
  line L298 (328.2476, 258.4329) -> (328.2434, 258.3962)
  line L299 (393.47, 247.2345) -> (392.9975, 247.4845)
  arc A230 (356.2056, 246.5924) -> (356.2176, 246.9165) centre (356.0214, 246.7615) ccw
  line L300 (377.3216, 272.3225) -> (377.3435, 271.7805)
  line L301 (391.2821, 244.7185) -> (391.2571, 244.6968)
  arc A231 (379.0489, 272.1174) -> (378.867, 272.0911) centre (381.1421, 257.037) ccw
  line L302 (356.4633, 247.2252) -> (356.1928, 247.3683)
  line L303 (360.0898, 257.5331) -> (360.0917, 257.5)
  line L304 (360.0904, 256.5508) -> (360.0925, 256.5878)
  line L305 (392.6202, 245.9547) -> (392.5978, 245.9303)
  arc A232 (355.2645, 245.8846) -> (355.59, 245.9218) centre (355.4058, 246.0908) ccw
  arc A233 (356.4633, 247.2252) -> (356.7824, 247.2992) centre (356.5802, 247.4461) ccw
  line L306 (328.4068, 257.7328) -> (328.7098, 257.776)
  line L307 (359.9293, 259.3478) -> (359.786, 260.1756)
  arc A234 (357.5014, 248.6936) -> (357.8101, 248.8035) centre (357.5924, 248.9265) ccw
  line L308 (390.6115, 244.4444) -> (390.3804, 244.9351)
  line L309 (396.0446, 262.1516) -> (395.5065, 262.0834)
  line L310 (393.8087, 247.3353) -> (394.2958, 248.0057)
  arc A235 (353.9207, 244.6894) -> (354.2484, 244.6893) centre (354.0846, 244.8782) ccw
  line L311 (359.563, 261.1323) -> (359.5723, 261.1005)
  arc A236 (377.5218, 272.5776) -> (377.3216, 272.3225) centre (377.5714, 272.3326) ccw
  arc A237 (357.3175, 248.0357) -> (357.2925, 248.3589) centre (357.1153, 248.1826) ccw
  line L312 (359.8967, 256.8462) -> (359.5916, 256.9133)
  arc A238 (357.0722, 248.5803) -> (357.2164, 248.805) centre (344.1421, 257.037) ccw
  line L313 (395.9026, 262.532) -> (395.4445, 262.2565)
  line L314 (360.0418, 258.3719) -> (360.0397, 258.4089)
  line L315 (376.5972, 272.3311) -> (376.6287, 272.3413)
  line L316 (391.2821, 244.7185) -> (391.9084, 245.2612)
  line L317 (396.5598, 261.1434) -> (396.3263, 261.9385)
  arc A239 (379.3169, 272.889) -> (379.0889, 272.6584) centre (379.3382, 272.6399) ccw
  line L318 (392.6202, 245.9547) -> (393.1805, 246.5652)
  line L319 (393.1805, 246.5652) -> (393.2056, 246.5924)
  line L320 (328.1921, 257.4522) -> (328.1921, 257.4853)
  line L321 (328.7007, 261.054) -> (328.7082, 261.0863)
  line L322 (377.5581, 272.5849) -> (377.5218, 272.5776)
  line L323 (359.786, 260.1756) -> (359.7797, 260.2121)
  line L324 (375.2484, 242.4252) -> (375.5493, 242.8765)
  line L325 (396.3263, 261.9385) -> (396.3159, 261.974)
  line L326 (392.2723, 245.8931) -> (391.8313, 246.1954)
  line L327 (390.9294, 244.697) -> (390.5258, 245.0476)
  line L328 (391.9084, 245.2612) -> (391.9363, 245.2854)
  arc A240 (376.9304, 272.2136) -> (376.6287, 272.3413) centre (376.7059, 272.1036) ccw
  line L329 (391.9852, 245.6059) -> (391.6997, 246.0671)
  line L330 (356.8019, 247.326) -> (357.2958, 248.0057)
  line L331 (376.5972, 272.3311) -> (375.8091, 272.075)
  line L332 (360.0898, 257.5331) -> (360.0418, 258.3719)
  line L333 (359.4361, 260.8026) -> (359.1575, 260.6758)
  line L334 (329.6411, 263.6931) -> (329.6248, 263.6599)
  arc A241 (354.9363, 245.2854) -> (354.9852, 245.6059) centre (354.7726, 245.4743) ccw
  line L335 (375.6289, 242.2833) -> (375.7207, 242.81)
  line L336 (394.2958, 248.0057) -> (394.3175, 248.0357)
  line L337 (378.3702, 272.7495) -> (378.4027, 272.7561)
  line L338 (328.5126, 253.8288) -> (328.5051, 253.861)
  arc A242 (332.0871, 246.5828) -> (332.4061, 246.5248) centre (332.2806, 246.741) ccw
  line L339 (328.9802, 252.0681) -> (329.2625, 251.2767)
  line L340 (328.5126, 253.8288) -> (328.7029, 253.0104)
  line L341 (330.0161, 249.6181) -> (330.0325, 249.5849)
  line L342 (328.9802, 252.0681) -> (328.9691, 252.0993)
  arc A243 (333.3573, 245.2768) -> (333.6809, 245.2555) centre (333.5316, 245.456) ccw
  line L343 (335.092, 244.1398) -> (335.3197, 244.3537)
  arc A244 (338.4217, 242.6851) -> (338.6705, 242.5884) centre (344.1421, 257.037) ccw
  arc A245 (337.9365, 242.3365) -> (338.2484, 242.4252) centre (338.0404, 242.5639) ccw
  line L344 (334.0735, 244.6597) -> (334.0473, 244.6799)
  line L345 (328.2488, 255.6313) -> (328.245, 255.6642)
  line L346 (331.5318, 247.2619) -> (331.5108, 247.2875)
  line L347 (329.556, 251.0801) -> (329.8631, 251.1369)
  line L348 (333.6809, 245.2555) -> (333.9314, 245.4421)
  line L349 (329.2625, 251.2767) -> (329.275, 251.2419)
  line L350 (333.9824, 245.0011) -> (334.1332, 245.2674)
  arc A246 (336.9725, 243.0127) -> (337.1085, 242.7146) centre (337.2123, 242.942) ccw
  arc A247 (336.3013, 243.1397) -> (336.6212, 243.1923) centre (336.4304, 243.3538) ccw
  line L351 (329.7143, 250.7187) -> (329.9671, 250.8911)
  arc A248 (334.7682, 244.124) -> (335.092, 244.1398) centre (334.9209, 244.322) ccw
  line L352 (328.2488, 255.6313) -> (328.3445, 254.7966)
  line L353 (339.6175, 241.7363) -> (339.6527, 241.7249)
  line L354 (333.3308, 245.3026) -> (333.3573, 245.2768)
  line L355 (332.0636, 246.6115) -> (332.0871, 246.5828)
  line L356 (332.4061, 246.5248) -> (332.6762, 246.6816)
  arc A249 (329.8631, 251.1369) -> (329.9671, 250.8911) centre (344.1421, 257.037) ccw
  arc A250 (329.7143, 250.7187) -> (329.6308, 250.4019) centre (329.8552, 250.5122) ccw
  line L357 (330.5286, 249.1152) -> (330.7601, 249.3154)
  line L358 (329.6454, 250.3721) -> (330.0161, 249.6181)
  line L359 (330.4997, 248.7631) -> (330.9539, 248.0563)
  arc A251 (330.5286, 249.1152) -> (330.4818, 248.7909) centre (330.6921, 248.9261) ccw
  line L360 (332.7282, 245.8881) -> (333.3308, 245.3026)
  line L361 (329.6454, 250.3721) -> (329.6308, 250.4019)
  line L362 (330.9539, 248.0563) -> (330.9739, 248.0251)
  line L363 (329.0881, 252.4045) -> (329.3589, 252.547)
  line L364 (331.5203, 247.615) -> (331.7275, 247.8403)
  line L365 (328.972, 252.7816) -> (329.2836, 252.8031)
  line L366 (328.6582, 254.1507) -> (328.9435, 254.2614)
  line L367 (331.2843, 247.9312) -> (331.5705, 248.0561)
  arc A252 (330.6287, 249.5477) -> (330.7601, 249.3154) centre (344.1421, 257.037) ccw
  line L368 (328.5858, 254.5386) -> (328.8978, 254.5244)
  line L369 (332.7282, 245.8881) -> (332.7045, 245.9112)
  line L370 (332.6766, 246.2377) -> (332.8568, 246.4851)
  line L371 (330.4997, 248.7631) -> (330.4818, 248.7909)
  line L372 (330.3301, 249.4562) -> (330.6287, 249.5477)
  line L373 (331.5318, 247.2619) -> (332.0636, 246.6115)
  line L374 (388.2285, 242.742) -> (388.1992, 242.7265)
  arc A253 (387.5342, 270.8552) -> (387.367, 270.9313) centre (381.1421, 257.037) ccw
  line L375 (387.325, 242.328) -> (387.3595, 242.3414)
  line L376 (351.9527, 270.95) -> (351.982, 270.9345)
  arc A254 (382.5189, 272.1997) -> (382.3358, 272.2152) centre (381.1421, 257.037) ccw
  arc A255 (338.2384, 271.6394) -> (337.924, 271.7319) centre (338.0279, 271.5045) ccw
  line L377 (354.2659, 269.3696) -> (354.238, 269.3938)
  line L378 (337.8939, 271.7181) -> (337.1297, 271.3691)
  arc A256 (385.7763, 242.5344) -> (385.951, 242.5914) centre (381.1421, 257.037) ccw
  line L379 (336.2611, 270.9102) -> (336.2895, 270.9273)
  arc A257 (335.0844, 269.9227) -> (334.7573, 269.9416) centre (334.91, 269.7436) ccw
  line L380 (352.4494, 243.6553) -> (352.2428, 243.881)
  line L381 (353.4877, 269.969) -> (352.7942, 270.4432)
  arc A258 (338.6522, 271.4787) -> (338.4035, 271.3817) centre (344.1421, 257.037) ccw
  line L382 (352.4412, 270.4299) -> (352.2261, 270.2033)
  arc A259 (387.3992, 243.1572) -> (387.5664, 243.2338) centre (381.1421, 257.037) ccw
  arc A260 (389.459, 243.6618) -> (389.7845, 243.6242) centre (389.6433, 243.8306) ccw
  line L383 (388.9614, 243.1287) -> (388.9941, 243.1459)
  line L384 (335.0844, 269.9227) -> (335.3036, 269.7092)
  line L385 (336.8058, 270.6341) -> (337.0417, 270.7588)
  line L386 (350.4994, 271.4477) -> (350.4297, 271.1497)
  arc A261 (352.7636, 270.4641) -> (352.4412, 270.4299) centre (352.6225, 270.2577) ccw
  line L387 (337.1297, 271.3691) -> (337.096, 271.3537)
  line L388 (389.8118, 243.6429) -> (389.7845, 243.6242)
  line L389 (389.459, 243.6618) -> (389.0979, 244.0561)
  line L390 (351.9527, 270.95) -> (351.2096, 271.3421)
  arc A262 (338.7739, 272.0636) -> (338.6041, 271.7874) centre (338.8511, 271.8258) ccw
  arc A263 (386.2134, 242.1256) -> (386.5219, 242.0153) centre (386.4312, 242.2483) ccw
  line L391 (352.8023, 243.6364) -> (352.7749, 243.6177)
  line L392 (353.4877, 269.969) -> (353.515, 269.9503)
  line L393 (350.8604, 271.2886) -> (350.6726, 271.039)
  line L394 (351.9614, 243.1287) -> (351.9941, 243.1459)
  line L395 (352.7942, 270.4432) -> (352.7636, 270.4641)
  arc A264 (351.1768, 271.3594) -> (350.8604, 271.2886) centre (351.0602, 271.1382) ccw
  line L396 (350.3158, 271.7496) -> (350.3467, 271.7376)
  arc A265 (350.6726, 271.039) -> (350.4297, 271.1497) centre (344.1421, 257.037) ccw
  arc A266 (337.096, 271.3537) -> (336.9588, 271.0599) centre (337.1998, 271.1263) ccw
  line L397 (352.1143, 243.4471) -> (352.0143, 243.743)
  line L398 (353.9137, 269.3965) -> (353.6743, 269.196)
  arc A267 (385.6438, 241.7285) -> (385.829, 241.9946) centre (385.5802, 241.9703) ccw
  line L399 (334.7311, 269.9214) -> (334.7573, 269.9416)
  arc A268 (384.2384, 271.9439) -> (384.0582, 271.9802) centre (381.1421, 257.037) ccw
  arc A269 (387.8801, 242.8009) -> (388.1992, 242.7265) centre (388.0825, 242.9476) ccw
  line L400 (350.5132, 242.6269) -> (350.4476, 242.9323)
  line L401 (389.1143, 243.4471) -> (388.9406, 243.961)
  line L402 (352.1007, 270.6291) -> (351.9975, 270.341)
  arc A270 (354.238, 269.3938) -> (353.9137, 269.3965) centre (354.0742, 269.2049) ccw
  line L403 (350.8699, 242.7955) -> (350.6903, 243.0433)
  arc A271 (385.9174, 271.4938) -> (385.7425, 271.5504) centre (381.1421, 257.037) ccw
  line L404 (351.2183, 242.7366) -> (351.189, 242.7211)
  line L405 (335.5416, 270.4763) -> (335.5099, 270.4572)
  arc A272 (387.3595, 242.3414) -> (387.5132, 242.6269) centre (387.2688, 242.5744) ccw
  line L406 (335.3036, 269.7092) -> (335.5239, 269.86)
  line L407 (388.2285, 242.742) -> (388.9614, 243.1287)
  line L408 (336.9588, 271.0599) -> (337.0417, 270.7588)
  line L409 (336.2611, 270.9102) -> (335.5416, 270.4763)
  line L410 (352.8023, 243.6364) -> (353.4958, 244.1107)
  line L411 (353.5982, 269.6333) -> (353.4628, 269.3589)
  line L412 (351.2183, 242.7366) -> (351.9614, 243.1287)
  line L413 (387.8801, 242.8009) -> (387.5664, 243.2338)
  line L414 (387.5132, 242.6269) -> (387.3992, 243.1572)
  line L415 (338.2384, 271.6394) -> (338.4035, 271.3817)
  arc A273 (388.9941, 243.1459) -> (389.1143, 243.4471) centre (388.8774, 243.3671) ccw
  line L416 (350.325, 242.328) -> (350.3595, 242.3414)
  line L417 (369.0636, 246.6115) -> (369.0871, 246.5828)
  line L418 (365.5104, 260.2357) -> (365.502, 260.1996)
  line L419 (389.7942, 270.4432) -> (389.7636, 270.4641)
  line L420 (368.2843, 247.9312) -> (368.7814, 248.1481)
  line L421 (365.5874, 259.5105) -> (366.1218, 259.5252)
  line L422 (338.6041, 271.7874) -> (338.6522, 271.4787)
  line L423 (389.4412, 270.4299) -> (389.0677, 270.0365)
  line L424 (365.9707, 261.2675) -> (366.5033, 261.2211)
  line L425 (367.9539, 248.0563) -> (367.9739, 248.0251)
  line L426 (367.5348, 249.1055) -> (367.9393, 249.4552)
  line L427 (386.5528, 242.0274) -> (387.325, 242.328)
  line L428 (351.2096, 271.3421) -> (351.1768, 271.3594)
  line L429 (366.2625, 251.2767) -> (366.275, 251.2419)
  line L430 (384.8065, 241.5084) -> (385.608, 241.7191)
  line L431 (365.1921, 257.4407) -> (365.1921, 257.4738)
  line L432 (334.7311, 269.9214) -> (334.0657, 269.4083)
  line L433 (365.6981, 261.0428) -> (365.7056, 261.0751)
  line L434 (389.0905, 270.6345) -> (388.9102, 270.1312)
  line L435 (366.6505, 250.3618) -> (367.0161, 249.6181)
  line L436 (367.5059, 248.7534) -> (367.9539, 248.0563)
  line L437 (336.6123, 270.8712) -> (336.8058, 270.6341)
  line L438 (366.2554, 262.7772) -> (365.9769, 261.9967)
  line L439 (366.0795, 261.6587) -> (366.5549, 261.3976)
  line L440 (385.829, 241.9946) -> (385.7763, 242.5344)
  line L441 (367.0161, 249.6181) -> (367.0325, 249.5849)
  line L442 (367.3301, 249.4562) -> (367.8487, 249.6151)
  arc A274 (390.5886, 269.6398) -> (390.5055, 269.9568) centre (390.3644, 269.7504) ccw
  line L443 (367.5059, 248.7534) -> (367.488, 248.7812)
  line L444 (366.6505, 250.3618) -> (366.6359, 250.3915)
  line L445 (366.7194, 250.7083) -> (367.161, 251.0096)
  line L446 (385.608, 241.7191) -> (385.6438, 241.7285)
  line L447 (390.4782, 269.9755) -> (389.7942, 270.4432)
  arc A275 (389.7636, 270.4641) -> (389.4412, 270.4299) centre (389.6225, 270.2577) ccw
  line L448 (354.9009, 268.8194) -> (354.2659, 269.3696)
  line L449 (388.9425, 270.9554) -> (388.9718, 270.9399)
  line L450 (365.3421, 259.2562) -> (365.3459, 259.2891)
  line L451 (365.4068, 257.7213) -> (365.9361, 257.7968)
  line L452 (339.6082, 272.3347) -> (338.8091, 272.075)
  line L453 (365.3421, 259.2562) -> (365.2476, 258.4329)
  line L454 (390.4782, 269.9755) -> (390.5055, 269.9568)
  line L455 (391.2659, 269.3696) -> (391.238, 269.3938)
  line L456 (335.4071, 270.1497) -> (335.5239, 269.86)
  line L457 (338.8091, 272.075) -> (338.7739, 272.0636)
  line L458 (366.556, 251.0801) -> (367.0893, 251.1788)
  line L459 (388.9425, 270.9554) -> (388.2096, 271.3421)
  arc A276 (390.4979, 269.0483) -> (390.3522, 269.1604) centre (381.1421, 257.037) ccw